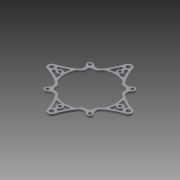
# Autodesk Inventor part: Center Plate
Saved by Autodesk Inventor 2014 SP1 (Build 180222100, 222)
## iProperties
Created: 2014-07-27
Part Number: Center Plate
Material: Generic
Document SubType Name: Modeling
Designer: Ryan
Density: 1 g/cm^3
Appearance: Default
Author: Ryan
Autodesk Inventor part; units mm, degrees
ref_plane "YZ Plane" through (0, 0, 0) normal (1, 0, 0) x (0, 1, 0)
ref_plane "XZ Plane" through (0, 0, 0) normal (0, 1, 0) x (-1, 0, 0)
ref_plane "XY Plane" through (0, 0, 0) normal (0, 0, 1) x (1, 0, 0)
sketch "Center Plate" plane through (0, 0, 0) normal (0, 0, 1) x (1, 0, 0)
  circle A0 centre (23.9383, 33.0301) radius 1.6
  circle A1 centre (23.9383, 78.0301) radius 1.6
  circle A2 centre (68.9383, 78.0301) radius 1.6
  circle A3 centre (68.9383, 33.0301) radius 1.6
  circle A4 centre (5.9467, 55.5301) radius 2.1
  circle A5 centre (86.93, 55.5301) radius 2.1
  circle A6 centre (46.4383, 96.0217) radius 2.1
  circle A7 centre (46.4383, 15.0384) radius 2.1
  arc A8 (50.2543, 97.2208) -> (42.6223, 97.2208) centre (46.4383, 96.0217) ccw
  arc A9 (4.9195, 59.3959) -> (4.9195, 51.6642) centre (5.9467, 55.5301) ccw
  arc A10 (4.9195, 59.3959) -> (21.6667, 67.9341) centre (-12.7128, 114.6743) ccw
  arc A11 (21.6667, 67.9341) -> (22.1885, 75.5478) centre (18.7041, 71.9619) ccw
  arc A12 (34.0449, 80.3186) -> (42.6223, 97.2208) centre (-12.7128, 114.6743) ccw
  arc A13 (26.5312, 79.6932) -> (34.0449, 80.3186) centre (30.0156, 83.2791) ccw
  arc A14 (42.6223, 13.8393) -> (50.2543, 13.8393) centre (46.4383, 15.0384) ccw
  arc A15 (42.6223, 13.8393) -> (34.0343, 30.7584) centre (-12.8047, -3.6558) ccw
  arc A16 (21.6498, 43.1366) -> (4.9195, 51.6642) centre (-12.6689, -3.518) ccw
  arc A17 (87.9571, 51.6642) -> (87.9571, 59.3959) centre (86.93, 55.5301) ccw
  arc A18 (50.2543, 97.2208) -> (58.8423, 80.3017) centre (105.6813, 114.7159) ccw
  arc A19 (71.2268, 67.9235) -> (87.9571, 59.3959) centre (105.5455, 114.5781) ccw
  arc A20 (87.9571, 51.6642) -> (71.21, 43.126) centre (105.5895, -3.6142) ccw
  arc A21 (58.8318, 30.7416) -> (50.2543, 13.8393) centre (105.5895, -3.6142) ccw
  line L0 (10.5293, 56.5301) -> (11.7901, 56.5301)
  line L1 (17.4469, 56.5301) -> (18.5189, 61.5546)
  arc A22 (9.7688, 59.1975) -> (17.0523, 62.6357) centre (-11.2986, 113.2601) ccw
  arc A23 (18.5189, 61.5546) -> (17.0523, 62.6357) centre (17.5409, 61.7632) ccw
  arc A24 (9.6127, 57.1301) -> (9.2948, 57.7186) centre (5.9467, 55.5301) ccw
  arc A25 (9.7688, 59.1975) -> (9.2948, 57.7186) centre (10.1319, 58.2658) ccw
  arc A26 (9.6127, 57.1301) -> (10.5293, 56.5301) centre (10.5293, 57.5301) ccw
  line L2 (10.5293, 54.5301) -> (11.7901, 54.5301)
  line L3 (17.4469, 54.5301) -> (18.5189, 49.5055)
  arc A27 (17.0523, 48.4244) -> (9.7688, 51.8626) centre (-11.2986, -2.2) ccw
  arc A28 (17.0523, 48.4244) -> (18.5189, 49.5055) centre (17.5409, 49.2969) ccw
  arc A29 (9.2948, 53.3415) -> (9.6127, 53.9301) centre (5.9467, 55.5301) ccw
  arc A30 (9.2948, 53.3415) -> (9.7688, 51.8626) centre (10.1319, 52.7944) ccw
  arc A31 (10.5293, 54.5301) -> (9.6127, 53.9301) centre (10.5293, 53.5301) ccw
  circle A32 centre (14.6185, 55.5301) radius 1.6
  circle A33 centre (46.4383, 87.3499) radius 1.6
  circle A34 centre (78.2581, 55.5301) radius 1.6
  circle A35 centre (46.4383, 23.7103) radius 1.6
  arc A36 (17.4469, 56.5301) -> (11.7901, 56.5301) centre (14.6185, 55.5301) ccw
  arc A37 (11.7901, 54.5301) -> (17.4469, 54.5301) centre (14.6185, 55.5301) ccw
  arc A38 (21.2966, 64.3013) -> (21.2966, 46.7589) centre (42.6725, 55.5301) ccw
  arc A39 (21.2966, 46.7589) -> (22.9693, 44.6221) centre (25.9223, 48.657) ccw
  arc A40 (22.9693, 66.438) -> (21.2966, 64.3013) centre (25.9223, 62.4032) ccw
  arc A41 (22.9693, 66.438) -> (24.3422, 67.4744) centre (-11.2986, 113.2601) ccw
  arc A42 (24.3422, 67.4744) -> (26.2479, 71.899) centre (21.2709, 71.4199) ccw
  arc A43 (34.4912, 77.6245) -> (35.5274, 78.9975) centre (-11.2986, 113.2601) ccw
  arc A44 (35.5304, 32.0611) -> (37.6638, 30.3897) centre (39.5317, 34.9713) ccw
  line L4 (82.3474, 56.5301) -> (81.0865, 56.5301)
  line L5 (75.4297, 56.5301) -> (74.3577, 61.5546)
  arc A45 (75.8244, 62.6357) -> (83.1078, 59.1975) centre (104.1752, 113.2601) ccw
  arc A46 (75.8244, 62.6357) -> (74.3577, 61.5546) centre (75.3357, 61.7632) ccw
  arc A47 (83.5818, 57.7186) -> (83.2639, 57.1301) centre (86.93, 55.5301) ccw
  arc A48 (83.5818, 57.7186) -> (83.1078, 59.1975) centre (82.7447, 58.2658) ccw
  arc A49 (82.3474, 56.5301) -> (83.2639, 57.1301) centre (82.3474, 57.5301) ccw
  line L6 (82.3474, 54.5301) -> (81.0865, 54.5301)
  line L7 (75.4297, 54.5301) -> (74.3577, 49.5055)
  arc A50 (83.1078, 51.8626) -> (75.8244, 48.4244) centre (104.1752, -2.2) ccw
  arc A51 (74.3577, 49.5055) -> (75.8244, 48.4244) centre (75.3357, 49.2969) ccw
  arc A52 (83.2639, 53.9301) -> (83.5818, 53.3415) centre (86.93, 55.5301) ccw
  arc A53 (83.1078, 51.8626) -> (83.5818, 53.3415) centre (82.7447, 52.7944) ccw
  arc A54 (83.2639, 53.9301) -> (82.3474, 54.5301) centre (82.3474, 53.5301) ccw
  arc A55 (81.0865, 56.5301) -> (75.4297, 56.5301) centre (78.2581, 55.5301) ccw
  arc A56 (75.4297, 54.5301) -> (81.0865, 54.5301) centre (78.2581, 55.5301) ccw
  arc A57 (71.5801, 46.7589) -> (71.5801, 64.3013) centre (50.2042, 55.5301) ccw
  arc A58 (69.9073, 44.6221) -> (71.5801, 46.7589) centre (66.9543, 48.657) ccw
  arc A59 (71.5801, 64.3013) -> (69.9032, 66.441) centre (66.9543, 62.4032) ccw
  line L8 (47.4383, 91.4391) -> (47.4383, 90.1783)
  line L9 (47.4383, 84.5214) -> (52.4628, 83.4495)
  arc A60 (50.1058, 92.1996) -> (53.544, 84.9161) centre (104.1683, 113.267) ccw
  arc A61 (52.4628, 83.4495) -> (53.544, 84.9161) centre (52.6715, 84.4275) ccw
  arc A62 (48.0383, 92.3556) -> (48.6269, 92.6735) centre (46.4383, 96.0217) ccw
  arc A63 (50.1058, 92.1996) -> (48.6269, 92.6735) centre (49.174, 91.8365) ccw
  arc A64 (48.0383, 92.3556) -> (47.4383, 91.4391) centre (48.4383, 91.4391) ccw
  line L10 (45.4383, 91.4391) -> (45.4383, 90.1783)
  line L11 (45.4383, 84.5214) -> (40.4138, 83.4495)
  arc A65 (39.3326, 84.9161) -> (42.7709, 92.1996) centre (-11.2917, 113.267) ccw
  arc A66 (39.3326, 84.9161) -> (40.4138, 83.4495) centre (40.2051, 84.4275) ccw
  arc A67 (44.2498, 92.6735) -> (44.8383, 92.3556) centre (46.4383, 96.0217) ccw
  arc A68 (44.2498, 92.6735) -> (42.7709, 92.1996) centre (43.7026, 91.8365) ccw
  arc A69 (45.4383, 91.4391) -> (44.8383, 92.3556) centre (44.4383, 91.4391) ccw
  arc A70 (47.4383, 84.5214) -> (47.4383, 90.1783) centre (46.4383, 87.3499) ccw
  arc A71 (45.4383, 90.1783) -> (45.4383, 84.5214) centre (46.4383, 87.3499) ccw
  arc A72 (55.2129, 80.6704) -> (37.6638, 80.6704) centre (46.4383, 59.2959) ccw
  arc A73 (37.6638, 80.6704) -> (35.5274, 78.9975) centre (39.5626, 76.045) ccw
  arc A74 (57.3492, 78.9975) -> (55.2129, 80.6704) centre (53.3141, 76.045) ccw
  line L12 (45.4383, 19.621) -> (45.4383, 20.8818)
  line L13 (45.4383, 26.5387) -> (40.4138, 27.6106)
  arc A75 (42.7709, 18.8605) -> (39.3326, 26.144) centre (-11.2917, -2.2069) ccw
  arc A76 (40.4138, 27.6106) -> (39.3326, 26.144) centre (40.2051, 26.6326) ccw
  arc A77 (44.8383, 18.7045) -> (44.2498, 18.3866) centre (46.4383, 15.0384) ccw
  arc A78 (42.7709, 18.8605) -> (44.2498, 18.3866) centre (43.7026, 19.2236) ccw
  arc A79 (44.8383, 18.7045) -> (45.4383, 19.621) centre (44.4383, 19.621) ccw
  line L14 (47.4383, 19.621) -> (47.4383, 20.8818)
  line L15 (47.4383, 26.5387) -> (52.4628, 27.6106)
  arc A80 (53.544, 26.144) -> (50.1058, 18.8605) centre (104.1683, -2.2069) ccw
  arc A81 (53.544, 26.144) -> (52.4628, 27.6106) centre (52.6715, 26.6326) ccw
  arc A82 (48.6269, 18.3866) -> (48.0383, 18.7045) centre (46.4383, 15.0384) ccw
  arc A83 (48.6269, 18.3866) -> (50.1058, 18.8605) centre (49.174, 19.2236) ccw
  arc A84 (47.4383, 19.621) -> (48.0383, 18.7045) centre (48.4383, 19.621) ccw
  arc A85 (45.4383, 26.5387) -> (45.4383, 20.8818) centre (46.4383, 23.7103) ccw
  arc A86 (47.4383, 20.8818) -> (47.4383, 26.5387) centre (46.4383, 23.7103) ccw
  arc A87 (37.6638, 30.3897) -> (55.2129, 30.3897) centre (46.4383, 51.7642) ccw
  arc A88 (55.2129, 30.3897) -> (57.3492, 32.0626) centre (53.3141, 35.0151) ccw
  arc A89 (26.0596, 80.1514) -> (21.8788, 75.8487) centre (23.9383, 78.0301) ccw
  line L16 (26.5312, 79.6932) -> (26.0596, 80.1514)
  line L17 (22.1885, 75.5478) -> (21.8788, 75.8487)
  arc A90 (30.0668, 75.7183) -> (26.2479, 71.899) centre (29.7318, 72.2344) ccw
  arc A91 (30.0668, 75.7183) -> (34.4912, 77.6245) centre (30.5453, 80.6954) ccw
  arc A92 (34.0343, 30.7584) -> (26.4206, 31.2802) centre (30.0065, 27.7958) ccw
  arc A93 (22.2752, 35.6229) -> (21.6498, 43.1366) centre (18.6893, 39.1073) ccw
  arc A94 (35.5304, 32.0611) -> (34.494, 33.4339) centre (-11.2917, -2.2069) ccw
  arc A95 (34.494, 33.4339) -> (30.0694, 35.3396) centre (30.5485, 30.3626) ccw
  arc A96 (24.3438, 43.5829) -> (22.9693, 44.6221) centre (-22.558, -17.0254) ccw
  arc A97 (21.817, 35.1514) -> (26.1197, 30.9705) centre (23.9383, 33.0301) ccw
  line L18 (22.2752, 35.6229) -> (21.817, 35.1514)
  line L19 (26.4206, 31.2802) -> (26.1197, 30.9705)
  arc A98 (26.25, 39.1585) -> (30.0694, 35.3396) centre (29.734, 38.8235) ccw
  arc A99 (26.25, 39.1585) -> (24.3438, 43.5829) centre (21.273, 39.6371) ccw
  arc A100 (58.8423, 80.3017) -> (66.456, 79.7799) centre (62.8701, 83.2643) ccw
  arc A101 (70.6014, 75.4372) -> (71.2268, 67.9235) centre (74.1874, 71.9528) ccw
  arc A102 (57.3492, 78.9975) -> (58.3826, 77.6262) centre (99.3198, 109.5501) ccw
  arc A103 (58.3826, 77.6262) -> (62.8073, 75.7205) centre (62.3281, 80.6975) ccw
  arc A104 (68.5328, 67.4772) -> (69.9032, 66.441) centre (108.8755, 119.4089) ccw
  arc A105 (71.0596, 75.9087) -> (66.757, 80.0896) centre (68.9383, 78.0301) ccw
  line L20 (70.6014, 75.4372) -> (71.0596, 75.9087)
  line L21 (66.456, 79.7799) -> (66.757, 80.0896)
  arc A106 (66.6266, 71.9016) -> (62.8073, 75.7205) centre (63.1427, 72.2366) ccw
  arc A107 (66.6266, 71.9016) -> (68.5328, 67.4772) centre (71.6036, 71.4231) ccw
  arc A108 (71.21, 43.126) -> (70.6882, 35.5123) centre (74.1726, 39.0983) ccw
  arc A109 (66.3455, 31.3669) -> (58.8318, 30.7416) centre (62.861, 27.781) ccw
  arc A110 (69.9073, 44.6221) -> (68.5345, 43.5858) centre (105.2854, -3.6706) ccw
  arc A111 (68.5345, 43.5858) -> (66.6288, 39.1611) centre (71.6058, 39.6402) ccw
  arc A112 (58.3854, 33.4356) -> (57.3492, 32.0626) centre (104.2014, -2.2197) ccw
  arc A113 (66.817, 30.9087) -> (70.9979, 35.2114) centre (68.9383, 33.0301) ccw
  line L22 (66.3455, 31.3669) -> (66.817, 30.9087)
  line L23 (70.6882, 35.5123) -> (70.9979, 35.2114)
  arc A114 (62.8099, 35.3418) -> (66.6288, 39.1611) centre (63.1449, 38.8257) ccw
  arc A115 (62.8099, 35.3418) -> (58.3854, 33.4356) centre (62.3313, 30.3647) ccw
  point P0 (46.4222, 55.5083)
sketch "Sketch1" plane through (0, 0, 0) normal (0, 1, 0) x (-1, 0, 0)
  circle A0 centre (5.9467, 55.5301) radius 2.1
  circle A1 centre (14.6185, 55.5301) radius 1.6
  circle A2 centre (23.9383, 78.0301) radius 1.6
  arc A3 (26.0596, 80.1514) -> (21.8788, 75.8487) centre (23.9383, 78.0301) ccw
  circle A4 centre (46.4383, 87.3499) radius 1.6
  circle A5 centre (46.4383, 96.0217) radius 2.1
  circle A6 centre (68.9383, 78.0301) radius 1.6
  circle A7 centre (78.2581, 55.5301) radius 1.6
  circle A8 centre (86.93, 55.5301) radius 2.1
  circle A9 centre (68.9383, 33.0301) radius 1.6
  arc A10 (66.817, 30.9087) -> (70.9979, 35.2114) centre (68.9383, 33.0301) ccw
  circle A11 centre (46.4383, 23.7103) radius 1.6
  circle A12 centre (46.4383, 15.0384) radius 2.1
  circle A13 centre (23.9383, 33.0301) radius 1.6
  arc A14 (47.4383, 84.5214) -> (47.4383, 90.1783) centre (46.4383, 87.3499) ccw
  arc A15 (45.4383, 90.1783) -> (45.4383, 84.5214) centre (46.4383, 87.3499) ccw
  arc A16 (48.0383, 92.3556) -> (48.6269, 92.6735) centre (46.4383, 96.0217) ccw
  arc A17 (44.2498, 92.6735) -> (44.8383, 92.3556) centre (46.4383, 96.0217) ccw
  arc A18 (50.2543, 97.2208) -> (42.6223, 97.2208) centre (46.4383, 96.0217) ccw
  arc A19 (81.0865, 56.5301) -> (75.4297, 56.5301) centre (78.2581, 55.5301) ccw
  arc A20 (75.4297, 54.5301) -> (81.0865, 54.5301) centre (78.2581, 55.5301) ccw
  arc A21 (83.2639, 53.9301) -> (83.5818, 53.3415) centre (86.93, 55.5301) ccw
  arc A22 (87.9571, 51.6642) -> (87.9571, 59.3959) centre (86.93, 55.5301) ccw
  arc A23 (83.5818, 57.7186) -> (83.2639, 57.1301) centre (86.93, 55.5301) ccw
  arc A24 (47.4383, 20.8818) -> (47.4383, 26.5387) centre (46.4383, 23.7103) ccw
  arc A25 (45.4383, 26.5387) -> (45.4383, 20.8818) centre (46.4383, 23.7103) ccw
  arc A26 (44.8383, 18.7045) -> (44.2498, 18.3866) centre (46.4383, 15.0384) ccw
  arc A27 (48.6269, 18.3866) -> (48.0383, 18.7045) centre (46.4383, 15.0384) ccw
  arc A28 (42.6223, 13.8393) -> (50.2543, 13.8393) centre (46.4383, 15.0384) ccw
  arc A29 (17.4469, 56.5301) -> (11.7901, 56.5301) centre (14.6185, 55.5301) ccw
  arc A30 (11.7901, 54.5301) -> (17.4469, 54.5301) centre (14.6185, 55.5301) ccw
  arc A31 (9.2948, 53.3415) -> (9.6127, 53.9301) centre (5.9467, 55.5301) ccw
  arc A32 (9.6127, 57.1301) -> (9.2948, 57.7186) centre (5.9467, 55.5301) ccw
  arc A33 (4.9195, 59.3959) -> (4.9195, 51.6642) centre (5.9467, 55.5301) ccw
  arc A34 (24.3422, 67.4744) -> (26.2479, 71.899) centre (21.2709, 71.4199) ccw
  arc A35 (21.6667, 67.9341) -> (22.1885, 75.5478) centre (18.7041, 71.9619) ccw
  line L0 (21.8788, 75.8487) -> (22.1885, 75.5478)
  arc A36 (30.0668, 75.7183) -> (34.4912, 77.6245) centre (30.5453, 80.6954) ccw
  arc A37 (26.5312, 79.6932) -> (34.0449, 80.3186) centre (30.0156, 83.2791) ccw
  line L1 (26.0596, 80.1514) -> (26.5312, 79.6932)
  arc A38 (57.3624, 78.9795) -> (55.2129, 80.6704) centre (53.3141, 76.045) ccw
  line L2 (57.3624, 78.9795) -> (58.3826, 77.6262)
  arc A39 (58.2896, 77.7496) -> (62.8073, 75.7205) centre (62.3281, 80.6975) ccw
  arc A40 (58.8406, 80.304) -> (66.456, 79.7799) centre (62.8701, 83.2643) ccw
  arc A41 (66.6266, 71.9016) -> (68.5365, 67.4743) centre (71.6036, 71.4231) ccw
  arc A42 (68.5364, 43.5873) -> (66.6288, 39.1611) centre (71.6058, 39.6402) ccw
  arc A43 (71.21, 43.126) -> (70.6882, 35.5123) centre (74.1726, 39.0983) ccw
  arc A44 (66.3455, 31.3669) -> (58.8318, 30.7416) centre (62.861, 27.781) ccw
  arc A45 (70.6014, 75.4372) -> (71.2244, 67.9253) centre (74.1874, 71.9528) ccw
  arc A46 (34.494, 33.4339) -> (30.0694, 35.3396) centre (30.5485, 30.3626) ccw
  arc A47 (34.036, 30.7561) -> (26.4206, 31.2802) centre (30.0065, 27.7958) ccw
  arc A48 (26.25, 39.1585) -> (24.3206, 43.6009) centre (21.273, 39.6371) ccw
  arc A49 (26.25, 39.1585) -> (30.0694, 35.3396) centre (29.734, 38.8235) ccw
  arc A50 (62.6894, 35.3519) -> (66.6186, 39.2815) centre (63.1449, 38.8257) ccw
  arc A51 (30.0668, 75.7183) -> (26.2479, 71.899) centre (29.7318, 72.2344) ccw
  arc A52 (66.6266, 71.9016) -> (62.8073, 75.7205) centre (63.1427, 72.2366) ccw
  arc A53 (22.2752, 35.6229) -> (21.6522, 43.1349) centre (18.6893, 39.1073) ccw
  line L3 (66.3455, 31.3669) -> (66.817, 30.9087)
  line L4 (70.6882, 35.5123) -> (70.9979, 35.2114)
  arc A54 (17.0523, 48.4244) -> (18.5189, 49.5055) centre (17.5409, 49.2969) ccw
  arc A55 (18.5189, 61.5546) -> (17.0523, 62.6357) centre (17.5409, 61.7632) ccw
  arc A56 (9.6127, 57.1301) -> (10.5293, 56.5301) centre (10.5293, 57.5301) ccw
  arc A57 (9.7688, 59.1975) -> (9.2948, 57.7186) centre (10.1319, 58.2658) ccw
  arc A58 (10.5293, 54.5301) -> (9.6127, 53.9301) centre (10.5293, 53.5301) ccw
  arc A59 (9.2948, 53.3415) -> (9.7688, 51.8626) centre (10.1319, 52.7944) ccw
  line L5 (17.4469, 56.5301) -> (18.5189, 61.5546)
  line L6 (11.7901, 56.5301) -> (10.5293, 56.5301)
  arc A60 (9.7688, 59.1975) -> (17.0523, 62.6357) centre (-11.2986, 113.2601) ccw
  arc A61 (17.0523, 48.4244) -> (9.7688, 51.8626) centre (-11.2986, -2.2) ccw
  line L7 (17.4469, 54.5301) -> (18.5189, 49.5055)
  line L8 (10.5293, 54.5301) -> (11.7901, 54.5301)
  arc A62 (4.9195, 59.3959) -> (21.6667, 67.9341) centre (-12.7128, 114.6743) ccw
  arc A63 (21.6522, 43.1349) -> (4.9195, 51.6642) centre (-12.6689, -3.518) ccw
  arc A64 (34.0449, 80.3186) -> (42.6223, 97.2208) centre (-12.7128, 114.6743) ccw
  arc A65 (87.9571, 51.6642) -> (71.21, 43.126) centre (105.5895, -3.6142) ccw
  arc A66 (58.8318, 30.7416) -> (50.2543, 13.8393) centre (105.5895, -3.6142) ccw
  arc A67 (42.6223, 13.8393) -> (34.036, 30.7561) centre (-12.8047, -3.6558) ccw
  arc A68 (39.3326, 84.9161) -> (40.4138, 83.4495) centre (40.2051, 84.4275) ccw
  arc A69 (52.4628, 83.4495) -> (53.544, 84.9161) centre (52.6715, 84.4275) ccw
  arc A70 (48.0383, 92.3556) -> (47.4383, 91.4391) centre (48.4383, 91.4391) ccw
  arc A71 (44.2498, 92.6735) -> (42.7709, 92.1996) centre (43.7026, 91.8365) ccw
  arc A72 (50.1058, 92.1996) -> (48.6269, 92.6735) centre (49.174, 91.8365) ccw
  arc A73 (45.4383, 91.4391) -> (44.8383, 92.3556) centre (44.4383, 91.4391) ccw
  line L9 (47.4383, 90.1783) -> (47.4383, 91.4391)
  line L10 (45.4383, 90.1783) -> (45.4383, 91.4391)
  line L11 (45.4383, 84.5214) -> (40.4138, 83.4495)
  line L12 (47.4383, 84.5214) -> (52.4628, 83.4495)
  arc A74 (39.3326, 84.9161) -> (42.7709, 92.1996) centre (-11.2917, 113.267) ccw
  arc A75 (50.1058, 92.1996) -> (53.544, 84.9161) centre (104.1683, 113.267) ccw
  arc A76 (75.8244, 62.6357) -> (74.3577, 61.5546) centre (75.3357, 61.7632) ccw
  arc A77 (82.3474, 56.5301) -> (83.2639, 57.1301) centre (82.3474, 57.5301) ccw
  arc A78 (83.5818, 57.7186) -> (83.1078, 59.1975) centre (82.7447, 58.2658) ccw
  arc A79 (83.2639, 53.9301) -> (82.3474, 54.5301) centre (82.3474, 53.5301) ccw
  arc A80 (83.1078, 51.8626) -> (83.5818, 53.3415) centre (82.7447, 52.7944) ccw
  arc A81 (74.3577, 49.5055) -> (75.8244, 48.4244) centre (75.3357, 49.2969) ccw
  line L13 (81.0865, 56.5301) -> (82.3474, 56.5301)
  line L14 (75.4297, 56.5301) -> (74.3577, 61.5546)
  line L15 (81.0865, 54.5301) -> (82.3474, 54.5301)
  line L16 (74.3577, 49.5055) -> (75.4297, 54.5301)
  arc A82 (83.1078, 51.8626) -> (75.8244, 48.4244) centre (104.1752, -2.2) ccw
  arc A83 (75.8244, 62.6357) -> (83.1078, 59.1975) centre (104.1752, 113.2601) ccw
  arc A84 (44.8383, 18.7045) -> (45.4383, 19.621) centre (44.4383, 19.621) ccw
  arc A85 (42.7709, 18.8605) -> (44.2498, 18.3866) centre (43.7026, 19.2236) ccw
  arc A86 (47.4383, 19.621) -> (48.0383, 18.7045) centre (48.4383, 19.621) ccw
  arc A87 (48.6269, 18.3866) -> (50.1058, 18.8605) centre (49.174, 19.2236) ccw
  arc A88 (40.4138, 27.6106) -> (39.3326, 26.144) centre (40.2051, 26.6326) ccw
  arc A89 (53.544, 26.144) -> (52.4628, 27.6106) centre (52.6715, 26.6326) ccw
  line L17 (40.4138, 27.6106) -> (45.4383, 26.5387)
  line L18 (47.4383, 26.5387) -> (52.4628, 27.6106)
  line L19 (47.4383, 20.8818) -> (47.4383, 19.621)
  line L20 (45.4383, 20.8818) -> (45.4383, 19.621)
  arc A90 (42.7709, 18.8605) -> (39.3326, 26.144) centre (-11.2917, -2.2069) ccw
  arc A91 (53.544, 26.144) -> (50.1058, 18.8605) centre (104.1683, -2.2069) ccw
  arc A92 (35.5304, 32.0611) -> (37.6638, 30.3897) centre (39.5317, 34.9713) ccw
  arc A93 (37.6638, 30.3897) -> (55.2129, 30.3897) centre (46.4383, 51.7642) ccw
  arc A94 (35.5304, 32.0611) -> (34.494, 33.4339) centre (-11.2917, -2.2069) ccw
  arc A95 (55.2129, 30.3897) -> (57.3492, 32.0626) centre (53.3141, 35.0151) ccw
  arc A96 (37.6638, 80.6704) -> (35.5274, 78.9975) centre (39.5626, 76.045) ccw
  arc A97 (55.2129, 80.6704) -> (37.6638, 80.6704) centre (46.4383, 59.2959) ccw
  arc A98 (34.4912, 77.6245) -> (35.5274, 78.9975) centre (-11.2986, 113.2601) ccw
  arc A99 (21.2966, 46.7589) -> (22.9693, 44.6221) centre (25.9223, 48.657) ccw
  arc A100 (22.9693, 66.438) -> (21.2966, 64.3013) centre (25.9223, 62.4032) ccw
  arc A101 (71.5801, 64.3013) -> (69.9032, 66.441) centre (66.9543, 62.4032) ccw
  arc A102 (24.3206, 43.6009) -> (22.9693, 44.6221) centre (-22.558, -17.0254) ccw
  arc A103 (21.2966, 64.3013) -> (21.2966, 46.7589) centre (42.6725, 55.5301) ccw
  arc A104 (22.9693, 66.438) -> (24.3422, 67.4744) centre (-11.2986, 113.2601) ccw
  arc A105 (68.5365, 67.4743) -> (69.9032, 66.441) centre (108.8822, 119.4178) ccw
  arc A106 (69.9073, 44.6221) -> (68.5364, 43.5873) centre (105.2874, -3.6732) ccw
  arc A107 (71.5801, 46.7589) -> (71.5801, 64.3013) centre (50.2042, 55.5301) ccw
  arc A108 (69.9073, 44.6221) -> (71.5801, 46.7589) centre (66.9543, 48.657) ccw
  line L21 (74.3577, 61.5546) -> (75.4297, 56.5301)
  arc A109 (81.0865, 56.5301) -> (75.4297, 56.5301) centre (78.2581, 55.5301) ccw
  arc A110 (82.3474, 56.5301) -> (83.2639, 57.1301) centre (82.3474, 57.5301) ccw
  arc A111 (83.5818, 57.7186) -> (83.2639, 57.1301) centre (86.93, 55.5301) ccw
  arc A112 (83.5818, 57.7186) -> (83.1078, 59.1975) centre (82.7447, 58.2658) ccw
  arc A113 (75.8244, 62.6357) -> (83.1078, 59.1975) centre (104.1752, 113.2601) ccw
  arc A114 (75.8244, 62.6357) -> (74.3577, 61.5546) centre (75.3357, 61.7632) ccw
  line L22 (81.0865, 56.5301) -> (82.3474, 56.5301)
  arc A115 (62.6894, 35.3519) -> (60.3529, 34.9567) centre (62.3313, 30.3647) ccw
  arc A116 (60.3529, 34.9567) -> (58.3854, 33.4356) centre (62.3313, 30.3647) ccw
  arc A117 (58.3854, 33.4356) -> (57.3492, 32.0626) centre (104.2014, -2.2197) ccw
  arc A118 (21.817, 35.1514) -> (26.1197, 30.9705) centre (23.9383, 33.0301) ccw
  line L23 (26.1197, 30.9705) -> (26.4206, 31.2802)
  line L24 (21.817, 35.1514) -> (22.2752, 35.6229)
  arc A119 (71.1197, 75.9705) -> (66.817, 80.1514) centre (68.9383, 78.0301) ccw
  line L25 (71.1197, 75.9705) -> (70.6014, 75.4372)
  line L26 (66.456, 79.7799) -> (66.817, 80.1514)
  arc A120 (50.2543, 97.2208) -> (58.8406, 80.304) centre (105.6813, 114.7159) ccw
  arc A121 (71.2244, 67.9253) -> (87.9571, 59.3959) centre (105.5455, 114.5781) ccw
  circle A122 centre (23.9383, 33.0301) radius 1.6
  circle A123 centre (23.9383, 78.0301) radius 1.6
  circle A124 centre (68.9383, 78.0301) radius 1.6
  circle A125 centre (68.9383, 33.0301) radius 1.6
  circle A126 centre (5.9467, 55.5301) radius 2.1
  circle A127 centre (86.93, 55.5301) radius 2.1
  circle A128 centre (46.4383, 96.0217) radius 2.1
  circle A129 centre (46.4383, 15.0384) radius 2.1
  arc A130 (50.2543, 97.2208) -> (42.6223, 97.2208) centre (46.4383, 96.0217) ccw
  arc A131 (4.9195, 59.3959) -> (4.9195, 51.6642) centre (5.9467, 55.5301) ccw
  arc A132 (4.9195, 59.3959) -> (21.6667, 67.9341) centre (-12.7128, 114.6743) ccw
  arc A133 (21.6667, 67.9341) -> (22.1885, 75.5478) centre (18.7041, 71.9619) ccw
  arc A134 (34.0449, 80.3186) -> (42.6223, 97.2208) centre (-12.7128, 114.6743) ccw
  arc A135 (26.5312, 79.6932) -> (34.0449, 80.3186) centre (30.0156, 83.2791) ccw
  arc A136 (42.6223, 13.8393) -> (50.2543, 13.8393) centre (46.4383, 15.0384) ccw
  arc A137 (42.6223, 13.8393) -> (34.0343, 30.7584) centre (-12.8047, -3.6558) ccw
  arc A138 (21.6498, 43.1366) -> (4.9195, 51.6642) centre (-12.6689, -3.518) ccw
  arc A139 (87.9571, 51.6642) -> (87.9571, 59.3959) centre (86.93, 55.5301) ccw
  arc A140 (50.2543, 97.2208) -> (58.8423, 80.3017) centre (105.6813, 114.7159) ccw
  arc A141 (71.2268, 67.9235) -> (87.9571, 59.3959) centre (105.5455, 114.5781) ccw
  arc A142 (87.9571, 51.6642) -> (71.21, 43.126) centre (105.5895, -3.6142) ccw
  arc A143 (58.8318, 30.7416) -> (50.2543, 13.8393) centre (105.5895, -3.6142) ccw
  line L27 (10.5293, 56.5301) -> (11.7901, 56.5301)
  line L28 (17.4469, 56.5301) -> (18.5189, 61.5546)
  arc A144 (9.7688, 59.1975) -> (17.0523, 62.6357) centre (-11.2986, 113.2601) ccw
  arc A145 (18.5189, 61.5546) -> (17.0523, 62.6357) centre (17.5409, 61.7632) ccw
  arc A146 (9.6127, 57.1301) -> (9.2948, 57.7186) centre (5.9467, 55.5301) ccw
  arc A147 (9.7688, 59.1975) -> (9.2948, 57.7186) centre (10.1319, 58.2658) ccw
  arc A148 (9.6127, 57.1301) -> (10.5293, 56.5301) centre (10.5293, 57.5301) ccw
  line L29 (10.5293, 54.5301) -> (11.7901, 54.5301)
  line L30 (17.4469, 54.5301) -> (18.5189, 49.5055)
  arc A149 (17.0523, 48.4244) -> (9.7688, 51.8626) centre (-11.2986, -2.2) ccw
  arc A150 (17.0523, 48.4244) -> (18.5189, 49.5055) centre (17.5409, 49.2969) ccw
  arc A151 (9.2948, 53.3415) -> (9.6127, 53.9301) centre (5.9467, 55.5301) ccw
  arc A152 (9.2948, 53.3415) -> (9.7688, 51.8626) centre (10.1319, 52.7944) ccw
  arc A153 (10.5293, 54.5301) -> (9.6127, 53.9301) centre (10.5293, 53.5301) ccw
  circle A154 centre (14.6185, 55.5301) radius 1.6
  circle A155 centre (46.4383, 87.3499) radius 1.6
  circle A156 centre (78.2581, 55.5301) radius 1.6
  circle A157 centre (46.4383, 23.7103) radius 1.6
  arc A158 (17.4469, 56.5301) -> (11.7901, 56.5301) centre (14.6185, 55.5301) ccw
  arc A159 (11.7901, 54.5301) -> (17.4469, 54.5301) centre (14.6185, 55.5301) ccw
  arc A160 (21.2966, 64.3013) -> (21.2966, 46.7589) centre (42.6725, 55.5301) ccw
  arc A161 (21.2966, 46.7589) -> (22.9693, 44.6221) centre (25.9223, 48.657) ccw
  arc A162 (22.9693, 66.438) -> (21.2966, 64.3013) centre (25.9223, 62.4032) ccw
  arc A163 (22.9693, 66.438) -> (24.3422, 67.4744) centre (-11.2986, 113.2601) ccw
  arc A164 (24.3422, 67.4744) -> (26.2479, 71.899) centre (21.2709, 71.4199) ccw
  arc A165 (34.4912, 77.6245) -> (35.5274, 78.9975) centre (-11.2986, 113.2601) ccw
  arc A166 (35.5304, 32.0611) -> (37.6638, 30.3897) centre (39.5317, 34.9713) ccw
  line L31 (82.3474, 56.5301) -> (81.0865, 56.5301)
  line L32 (75.4297, 56.5301) -> (74.3577, 61.5546)
  arc A167 (75.8244, 62.6357) -> (83.1078, 59.1975) centre (104.1752, 113.2601) ccw
  arc A168 (75.8244, 62.6357) -> (74.3577, 61.5546) centre (75.3357, 61.7632) ccw
  arc A169 (83.5818, 57.7186) -> (83.2639, 57.1301) centre (86.93, 55.5301) ccw
  arc A170 (83.5818, 57.7186) -> (83.1078, 59.1975) centre (82.7447, 58.2658) ccw
  arc A171 (82.3474, 56.5301) -> (83.2639, 57.1301) centre (82.3474, 57.5301) ccw
  line L33 (82.3474, 54.5301) -> (81.0865, 54.5301)
  line L34 (75.4297, 54.5301) -> (74.3577, 49.5055)
  arc A172 (83.1078, 51.8626) -> (75.8244, 48.4244) centre (104.1752, -2.2) ccw
  arc A173 (74.3577, 49.5055) -> (75.8244, 48.4244) centre (75.3357, 49.2969) ccw
  arc A174 (83.2639, 53.9301) -> (83.5818, 53.3415) centre (86.93, 55.5301) ccw
  arc A175 (83.1078, 51.8626) -> (83.5818, 53.3415) centre (82.7447, 52.7944) ccw
  arc A176 (83.2639, 53.9301) -> (82.3474, 54.5301) centre (82.3474, 53.5301) ccw
  arc A177 (81.0865, 56.5301) -> (75.4297, 56.5301) centre (78.2581, 55.5301) ccw
  arc A178 (75.4297, 54.5301) -> (81.0865, 54.5301) centre (78.2581, 55.5301) ccw
  arc A179 (71.5801, 46.7589) -> (71.5801, 64.3013) centre (50.2042, 55.5301) ccw
  arc A180 (69.9073, 44.6221) -> (71.5801, 46.7589) centre (66.9543, 48.657) ccw
  arc A181 (71.5801, 64.3013) -> (69.9032, 66.441) centre (66.9543, 62.4032) ccw
  line L35 (47.4383, 91.4391) -> (47.4383, 90.1783)
  line L36 (47.4383, 84.5214) -> (52.4628, 83.4495)
  arc A182 (50.1058, 92.1996) -> (53.544, 84.9161) centre (104.1683, 113.267) ccw
  arc A183 (52.4628, 83.4495) -> (53.544, 84.9161) centre (52.6715, 84.4275) ccw
  arc A184 (48.0383, 92.3556) -> (48.6269, 92.6735) centre (46.4383, 96.0217) ccw
  arc A185 (50.1058, 92.1996) -> (48.6269, 92.6735) centre (49.174, 91.8365) ccw
  arc A186 (48.0383, 92.3556) -> (47.4383, 91.4391) centre (48.4383, 91.4391) ccw
  line L37 (45.4383, 91.4391) -> (45.4383, 90.1783)
  line L38 (45.4383, 84.5214) -> (40.4138, 83.4495)
  arc A187 (39.3326, 84.9161) -> (42.7709, 92.1996) centre (-11.2917, 113.267) ccw
  arc A188 (39.3326, 84.9161) -> (40.4138, 83.4495) centre (40.2051, 84.4275) ccw
  arc A189 (44.2498, 92.6735) -> (44.8383, 92.3556) centre (46.4383, 96.0217) ccw
  arc A190 (44.2498, 92.6735) -> (42.7709, 92.1996) centre (43.7026, 91.8365) ccw
  arc A191 (45.4383, 91.4391) -> (44.8383, 92.3556) centre (44.4383, 91.4391) ccw
  arc A192 (47.4383, 84.5214) -> (47.4383, 90.1783) centre (46.4383, 87.3499) ccw
  arc A193 (45.4383, 90.1783) -> (45.4383, 84.5214) centre (46.4383, 87.3499) ccw
  arc A194 (55.2129, 80.6704) -> (37.6638, 80.6704) centre (46.4383, 59.2959) ccw
  arc A195 (37.6638, 80.6704) -> (35.5274, 78.9975) centre (39.5626, 76.045) ccw
  arc A196 (57.3492, 78.9975) -> (55.2129, 80.6704) centre (53.3141, 76.045) ccw
  line L39 (45.4383, 19.621) -> (45.4383, 20.8818)
  line L40 (45.4383, 26.5387) -> (40.4138, 27.6106)
  arc A197 (42.7709, 18.8605) -> (39.3326, 26.144) centre (-11.2917, -2.2069) ccw
  arc A198 (40.4138, 27.6106) -> (39.3326, 26.144) centre (40.2051, 26.6326) ccw
  arc A199 (44.8383, 18.7045) -> (44.2498, 18.3866) centre (46.4383, 15.0384) ccw
  arc A200 (42.7709, 18.8605) -> (44.2498, 18.3866) centre (43.7026, 19.2236) ccw
  arc A201 (44.8383, 18.7045) -> (45.4383, 19.621) centre (44.4383, 19.621) ccw
  line L41 (47.4383, 19.621) -> (47.4383, 20.8818)
  line L42 (47.4383, 26.5387) -> (52.4628, 27.6106)
  arc A202 (53.544, 26.144) -> (50.1058, 18.8605) centre (104.1683, -2.2069) ccw
  arc A203 (53.544, 26.144) -> (52.4628, 27.6106) centre (52.6715, 26.6326) ccw
  arc A204 (48.6269, 18.3866) -> (48.0383, 18.7045) centre (46.4383, 15.0384) ccw
  arc A205 (48.6269, 18.3866) -> (50.1058, 18.8605) centre (49.174, 19.2236) ccw
  arc A206 (47.4383, 19.621) -> (48.0383, 18.7045) centre (48.4383, 19.621) ccw
  arc A207 (45.4383, 26.5387) -> (45.4383, 20.8818) centre (46.4383, 23.7103) ccw
  arc A208 (47.4383, 20.8818) -> (47.4383, 26.5387) centre (46.4383, 23.7103) ccw
  arc A209 (37.6638, 30.3897) -> (55.2129, 30.3897) centre (46.4383, 51.7642) ccw
  arc A210 (55.2129, 30.3897) -> (57.3492, 32.0626) centre (53.3141, 35.0151) ccw
  arc A211 (26.0596, 80.1514) -> (21.8788, 75.8487) centre (23.9383, 78.0301) ccw
  line L43 (26.5312, 79.6932) -> (26.0596, 80.1514)
  line L44 (22.1885, 75.5478) -> (21.8788, 75.8487)
  arc A212 (30.0668, 75.7183) -> (26.2479, 71.899) centre (29.7318, 72.2344) ccw
  arc A213 (30.0668, 75.7183) -> (34.4912, 77.6245) centre (30.5453, 80.6954) ccw
  arc A214 (34.0343, 30.7584) -> (26.4206, 31.2802) centre (30.0065, 27.7958) ccw
  arc A215 (22.2752, 35.6229) -> (21.6498, 43.1366) centre (18.6893, 39.1073) ccw
  arc A216 (35.5304, 32.0611) -> (34.494, 33.4339) centre (-11.2917, -2.2069) ccw
  arc A217 (34.494, 33.4339) -> (30.0694, 35.3396) centre (30.5485, 30.3626) ccw
  arc A218 (24.3438, 43.5829) -> (22.9693, 44.6221) centre (-22.558, -17.0254) ccw
  arc A219 (21.817, 35.1514) -> (26.1197, 30.9705) centre (23.9383, 33.0301) ccw
  line L45 (22.2752, 35.6229) -> (21.817, 35.1514)
  line L46 (26.4206, 31.2802) -> (26.1197, 30.9705)
  arc A220 (26.25, 39.1585) -> (30.0694, 35.3396) centre (29.734, 38.8235) ccw
  arc A221 (26.25, 39.1585) -> (24.3438, 43.5829) centre (21.273, 39.6371) ccw
  arc A222 (58.8423, 80.3017) -> (66.456, 79.7799) centre (62.8701, 83.2643) ccw
  arc A223 (70.6014, 75.4372) -> (71.2268, 67.9235) centre (74.1874, 71.9528) ccw
  arc A224 (57.3492, 78.9975) -> (58.3826, 77.6262) centre (99.3198, 109.5501) ccw
  arc A225 (58.3826, 77.6262) -> (62.8073, 75.7205) centre (62.3281, 80.6975) ccw
  arc A226 (68.5328, 67.4772) -> (69.9032, 66.441) centre (108.8755, 119.4089) ccw
  arc A227 (71.0596, 75.9087) -> (66.757, 80.0896) centre (68.9383, 78.0301) ccw
  line L47 (70.6014, 75.4372) -> (71.0596, 75.9087)
  line L48 (66.456, 79.7799) -> (66.757, 80.0896)
  arc A228 (66.6266, 71.9016) -> (62.8073, 75.7205) centre (63.1427, 72.2366) ccw
  arc A229 (66.6266, 71.9016) -> (68.5328, 67.4772) centre (71.6036, 71.4231) ccw
  arc A230 (71.21, 43.126) -> (70.6882, 35.5123) centre (74.1726, 39.0983) ccw
  arc A231 (66.3455, 31.3669) -> (58.8318, 30.7416) centre (62.861, 27.781) ccw
  arc A232 (69.9073, 44.6221) -> (68.5345, 43.5858) centre (105.2854, -3.6706) ccw
  arc A233 (68.5345, 43.5858) -> (66.6288, 39.1611) centre (71.6058, 39.6402) ccw
  arc A234 (58.3854, 33.4356) -> (57.3492, 32.0626) centre (104.2014, -2.2197) ccw
  arc A235 (66.817, 30.9087) -> (70.9979, 35.2114) centre (68.9383, 33.0301) ccw
  line L49 (66.3455, 31.3669) -> (66.817, 30.9087)
  line L50 (70.6882, 35.5123) -> (70.9979, 35.2114)
  arc A236 (62.8099, 35.3418) -> (66.6288, 39.1611) centre (63.1449, 38.8257) ccw
  arc A237 (62.8099, 35.3418) -> (58.3854, 33.4356) centre (62.3313, 30.3647) ccw
  point P0 (0, 0)
  constraints: 221 point on circle, 122 centre point, 54 end point, 30 tangent, 10 coincident, 10 horizontal, 6 vertical, 3 concentric, 2 parallel, 1 perpendicular, 1 point on line, 280 other
extrude "Extrusion1" add sketch "Sketch1" along normal blind 2
body "Solid1"
